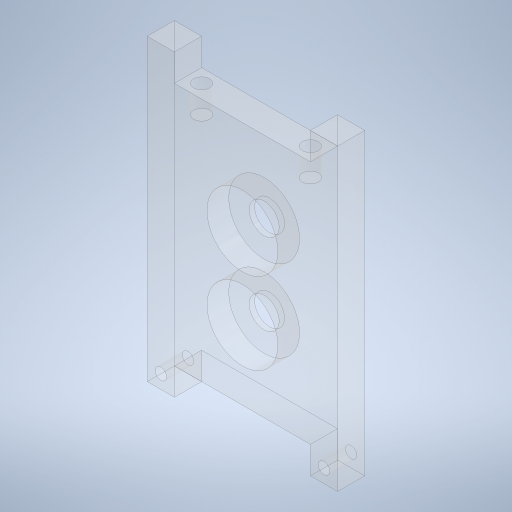
# Autodesk Inventor part: gearbox_side1
Saved by Autodesk Inventor 2023 (Build 270158000, 158)
## iProperties
Created: 2023-05-27
Part Number: gearbox_side1
Material: PMMA Plastic
Document SubType Name: Modeling
Designer: 310611102
Density: 1.13748 g/cm^3
Appearance: Polycarbonate - Clear
Mass: 65.2 g
Surface Area: 190.379 cm^2
Volume: 57.3195 cm^3
Vendor: 新采硯
Author: 310611102
Autodesk Inventor part; units mm, degrees
ref_plane "YZ Plane" through (0, 0, 0) normal (1, 0, 0) x (0, 1, 0)
ref_plane "XZ Plane" through (0, 0, 0) normal (0, 1, 0) x (-1, 0, 0)
ref_plane "XY Plane" through (0, 0, 0) normal (0, 0, 1) x (1, 0, 0)
sketch "Sketch1" plane through (0, 0, 0) normal (0, 0, 1) x (1, 0, 0)
  line L0 (-25, 45) -> (25, 45)
  line L1 (35, 44.3995) -> (35, -45)
  line L2 (25, -45) -> (-25, -45)
  line L3 (-35, -44.3995) -> (-35, 45)
  line L4 (-35, 45) -> (35, -45) construction
  line L5 (35, 44.3995) -> (-35, -44.3995) construction
  line L6 (-25, 55) -> (-35, 55)
  line L7 (-35, 55) -> (-35, 45)
  line L8 (-25, 45) -> (-25, 55)
  line L9 (-25, 55) -> (-35, 45) construction
  line L10 (-35, 55) -> (-25, 45) construction
  line L11 (0, 15.2738) -> (0, -11.5274)
  line L12 (-10.8069, 0) -> (18.2997, 0)
  line L13 (25, 55) -> (35, 55)
  line L14 (35, 55) -> (35, 44.3995)
  line L15 (25, 45) -> (25, 55)
  line L16 (25, 55) -> (35, 44.3995) construction
  line L17 (35, 55) -> (25, 45) construction
  line L18 (-25, -55) -> (-35, -55)
  line L19 (-35, -55) -> (-35, -44.3995)
  line L20 (-25, -45) -> (-25, -55)
  line L21 (-25, -55) -> (-35, -44.3995) construction
  line L22 (-35, -55) -> (-25, -45) construction
  line L23 (25, -55) -> (35, -55)
  line L24 (35, -55) -> (35, -45)
  line L25 (25, -45) -> (25, -55)
  line L26 (25, -55) -> (35, -45) construction
  line L27 (35, -55) -> (25, -45) construction
  point P0 (0, 0)
  point P1 (-30, 50)
  point P2 (30, 50)
  point P3 (-30, -50)
  point P4 (30, -50)
  dimension "d0" = 70
  dimension "d1" = 10
  dimension "d2" = 90
  constraints: 52 end point, 12 symmetric about line, 4 midpoint, 3 horizontal, 3 parallel, 3 perpendicular, 2 point on line, 1 vertical, 6 other
  measures "d0" distance between parallel lines of L3 L1
  measures "d1" distance of L6.start L6.end
  measures "d2" distance between parallel lines of L2 L0
extrude "Extrusion1" add sketch "Sketch1" along normal blind 10
sketch "Sketch2" plane through (0, 0, 10) normal (0, 0, 1) x (1, 0, 0)
  circle A0 centre (0, 10.48) radius 13
  circle A1 centre (0, -19.52) radius 13
  line L0 (-25, -45) -> (25, -45) projected
  line L1 (-35, -55) -> (-25, -55) projected
  point P0 (0, 0)
  dimension "d6" = 26
  dimension "d11" = 26
  dimension "d15" = 30
  dimension "d40" = 35.48
  constraints: 2 centre point, 2 vertical alignment, 1 other
  measures "d6" diameter of A0
  measures "d11" diameter of A1
  measures "d15" distance of A1.centre A0.centre
  measures "d40" distance from line of L1 A1.centre
extrude "Extrusion2" cut sketch "Sketch2" against normal blind 8
sketch "Sketch3" plane through (0, 10.48, 2) normal (0, 0, 1) x (1, 0, 0)
  circle A0 centre (0, 0) radius 5.5
  circle A1 centre (0, 0) radius 13 projected
  point P0 (0, -10.48)
  point P1 (-9.0139, 15)
  point P2 (9.0139, 15)
  dimension "d16" = 11
  constraints: 1 centre point, 2 other
  measures "d16" diameter of A0
extrude "Extrusion3" cut sketch "Sketch3" against normal through all contours A0
sketch "Sketch6" plane through (0, -19.52, 2) normal (0, 0, 1) x (1, 0, 0)
  circle A0 centre (0, 0) radius 5.5
  point P0 (0, 19.52)
  dimension "d19" = 11
  constraints: 1 centre point
  measures "d19" diameter of A0
extrude "Extrusion4" cut sketch "Sketch6" against normal blind 10
sketch "Sketch8" plane through (-25, 45, 0) normal (0, 1, 0) x (1, 0, 0)
  circle A0 centre (5, -5) radius 2.9
  line L0 (0, 0) -> (0, -10) projected
  line L1 (50, 0) -> (0, 0) projected
  circle A1 centre (45, -5) radius 2.9
  line L2 (50, 0) -> (50, -10) projected
  point P0 (25, 0)
  dimension "d30" = 5.8
  dimension "d31" = 5
  dimension "d32" = 5
  dimension "d33" = 5.8
  dimension "d34" = 5
  dimension "d35" = 5
  constraints: 2 centre point
  measures "d30" diameter of A0
  measures "d31" distance from line of L0 A0.centre
  measures "d32" distance from line of L1 A0.centre
  measures "d33" diameter of A1
  measures "d34" distance from line of L2 A1.centre
  measures "d35" distance from line of L1 A1.centre
extrude "Extrusion6" cut sketch "Sketch8" against normal blind 10
sketch "Sketch11" plane through (0, 0, 10) normal (0, 0, 1) x (1, 0, 0)
  line L0 (-35, 55) -> (-35, -55) projected
  line L1 (-25, 55) -> (-35, 55) projected
  line L2 (0, 0) -> (0, 27.2927)
  line L3 (0, 0) -> (14.8331, 0)
  circle A0 centre (-30, -50) radius 2.1
  circle A1 centre (30, -50) radius 2.1
  line L4 (-35, -55) -> (-25, -55) projected
  line L5 (25, -45) -> (25, -55) projected
  line L6 (25, -55) -> (35, -55) projected
  point P0 (30, -55)
  dimension "d54" = 4.2
  dimension "d55" = 5
  dimension "d56" = 5
  dimension "d57" = 4.2
  dimension "d58" = 5
  dimension "d59" = 5
  constraints: 4 end point, 2 centre point, 1 horizontal, 1 midpoint, 1 vertical
  measures "d54" diameter of A0
  measures "d55" distance from line of L0 A0.centre
  measures "d56" distance from line of L4 A0.centre
  measures "d57" diameter of A1
  measures "d58" distance from line of L5 A1.centre
  measures "d59" distance of point (30, -55) A1.centre
extrude "Extrusion9" cut sketch "Sketch11" against normal through all
sketch "Sketch7" plane through (0, -48, 10) normal (0, 0, -1) x (-1, 0, 0)
  circle A0 centre (0, 22.5) radius 1.6
  circle A1 centre (-22.5, 0) radius 1.6
  circle A2 centre (0, -22.5) radius 1.6
  circle A3 centre (22.5, 0) radius 1.6
  point P0 (0, 48)
  point P1 (0, 0)
  dimension "d22" = 3.2
  dimension "d25" = 360
  dimension "d27" = 45
  constraints: 4 centre point, 1 vertical alignment, 10 other
  measures "d22" diameter of A0
  measures "d27" distance of A2.centre A0.centre
equation "\"d33\" = d30"
equation "\"d57\" = d54"
equation "\"d58\" = d55"
equation "\"d59\" = d56"
body "Solid1"
